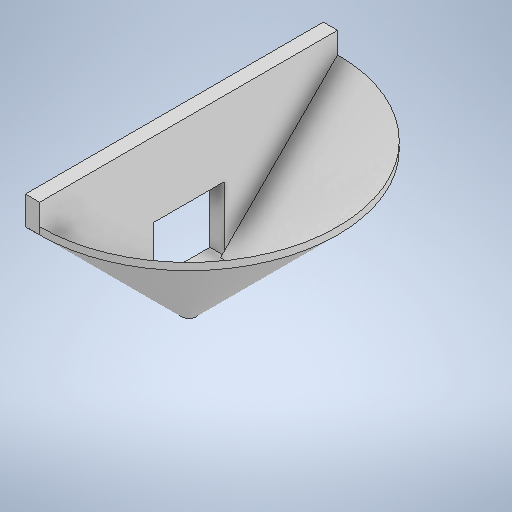
# Autodesk Inventor part: Collector
Saved by Autodesk Inventor 2025.3 (Build 293356000, 356)
## iProperties
Created: 2026-04-19
Part Number: Collector
Material: Generic
Document SubType Name: Modeling
Designer: kamal
Density: 1 g/cm^3
Appearance: Default
Author: kamal
Autodesk Inventor part; units mm, degrees
ref_plane "YZ Plane" through (0, 0, 0) normal (1, 0, 0) x (0, 1, 0)
ref_plane "XZ Plane" through (0, 0, 0) normal (0, 1, 0) x (-1, 0, 0)
sketch "Sketch1" plane through (0, 0, 0) normal (0, 0, 1) x (1, 0, 0)
  line L0 (0, 0) -> (5, 0)
  line L1 (5, 0) -> (105, 0)
  line L2 (105, 0) -> (105, 100)
  line L3 (105, 100) -> (5, 0)
  line L4 (0, 0) -> (105, 105)
  line L5 (105, 105) -> (105, 100)
  line L6 (0, 0) -> (0, 120) construction
  dimension "d0" = 5
  dimension "d1" = 100
  dimension "d2" = 100
  dimension "d3" = 120
  constraints: 14 end point, 2 point on line, 1 horizontal, 1 parallel, 1 perpendicular, 1 vertical
  measures "d0" distance of L0.start L0.end
  measures "d1" distance of L0.end L1.end
  measures "d2" distance of L1.end L2.end
  measures "d3" distance of L0.start L6.end
revolve "Revolution1" add sketch "Sketch1" angle 360 about axis through (0, 0, 0) along (0, 1, 0) contours L4 L5 L3 L0
ref_plane "Work Plane1" through (0, 0, 0) normal (0, 0, -1) x (0, 1, 0)
sketch "Sketch2" plane through (0, 0, 0) normal (0, 0, -1) x (0, 1, 0)
  line L0 (120, 0) -> (120, -10)
  line L1 (120, -10) -> (0, -10)
  line L2 (0, -10) -> (0, 0)
  line L3 (120, -10) -> (120, -110)
  line L4 (120, -110) -> (0, -110)
  line L5 (0, -110) -> (0, -10)
  line L6 (120, 0) -> (0, 0)
  dimension "d5" = 10
  dimension "d6" = 120
  dimension "d7" = 10
  dimension "d8" = 100
  constraints: 14 end point, 4 perpendicular, 2 vertical
  measures "d5" distance of L0.start L0.end
  measures "d6" distance between parallel lines of L0 L2
  measures "d7" distance from line of L2.end L1
  measures "d8" distance of L0.end L3.end
extrude "Extrusion1" cut sketch "Sketch2" along normal through all both and the other way through all contours L3 L4 L5 L1
extrude "Extrusion2" add sketch "Sketch2" along normal mid plane 210 contours L0 L1 L2 L6
sketch "Sketch3" plane through (0, 0, 105) normal (1, 0, 0) x (0, 0, -1)
  line L0 (0, 100) -> (100, 0) projected
  line L1 (0, 0) -> (0, 100) projected
  line L2 (100, 0) -> (0, 0) projected
  line L3 (110, 0) -> (210, 100) projected
  line L4 (210, 0) -> (110, 0) projected
  line L5 (210, 100) -> (210, 0) projected
  point P0 (105, 0)
extrude "Extrusion3" cut sketch "Sketch3" against normal through all
sketch "Sketch4" plane through (-10, 120, -105) normal (-1, 0, 0) x (0, 0, 1)
  line L0 (105, -120) -> (105, -75)
  line L1 (130, -52.5) -> (80, -52.5)
  line L2 (80, -52.5) -> (80, -97.5)
  line L3 (80, -97.5) -> (130, -97.5)
  line L4 (130, -97.5) -> (130, -52.5)
  line L5 (130, -52.5) -> (80, -97.5) construction
  line L6 (80, -52.5) -> (130, -97.5) construction
  dimension "d15" = 45
  dimension "d16" = 50
  dimension "d17" = 45
  constraints: 14 end point, 2 midpoint, 2 parallel, 1 horizontal, 1 perpendicular, 1 vertical
  measures "d15" distance of L0.start L0.end
  measures "d16" distance of L3.end L2.end
  measures "d17" distance of L2.end L1.end
extrude "Extrusion4" cut sketch "Sketch4" against normal blind 10
sketch "Sketch5" plane through (0, 22.5, 22.5) normal (1, 0, 0) x (0, 0, -1)
  line L0 (45, 0) -> (0, 0) projected
  line L1 (127.5, 82.5) -> (22.5, -22.5) projected
  line L2 (22.5, -22.5) -> (0, 0) projected
extrude "Extrusion5" add sketch "Sketch5" along normal blind 25
revolve "Revolution2" cut sketch "Sketch1" angle 360 about axis through (0, 0, 0) along (0, 1, 0) contours L3 L2 L1
body "Solid1"
